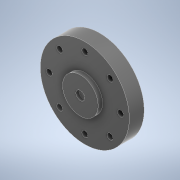
# Autodesk Inventor part: orczyk serwa okrągły 02-1
Saved by Autodesk Inventor 2021 (Build 250183000, 183)
## iProperties
Created: 2021-11-05
Part Number: orczyk serwa okrągły 02-1
Material: Generic
Document SubType Name: Modeling
Designer: Łukasz
Density: 1 g/cm^3
Appearance: Smooth - Black
Author: Łukasz
Autodesk Inventor part; units mm, degrees
ref_plane "YZ Plane" through (0, 0, 0) normal (1, 0, 0) x (0, 1, 0)
ref_plane "XZ Plane" through (0, 0, 0) normal (0, 1, 0) x (-1, 0, 0)
ref_plane "XY Plane" through (0, 0, 0) normal (0, 0, 1) x (1, 0, 0)
sketch "Sketch1" plane through (0, 0, 0) normal (0, 0, 1) x (1, 0, 0)
  circle A0 centre (0, 0) radius 15
  circle A1 centre (0, 12) radius 1
  circle A2 centre (-8.4853, 8.4853) radius 1
  circle A3 centre (-12, 0) radius 1
  circle A4 centre (-8.4853, -8.4853) radius 1
  circle A5 centre (0, -12) radius 1
  circle A6 centre (8.4853, -8.4853) radius 1
  circle A7 centre (12, 0) radius 1
  circle A8 centre (8.4853, 8.4853) radius 1
  circle A9 centre (0, 0) radius 1.5
  dimension "d0" = 30
  dimension "d1" = 2
  dimension "d4" = 360
  dimension "d6" = 12
  dimension "d9" = 3
  constraints: 10 centre point, 2 coincident, 17 other
  measures "d0" diameter of A0
  measures "d1" diameter of A1
  measures "d6" distance of point (0, 0) A1.centre
  measures "d9" diameter of A9
extrude "Extrusion1" add sketch "Sketch1" along normal blind 5
sketch "Sketch2" plane through (0, 0, 5) normal (0, 0, 1) x (1, 0, 0)
  point P0 (0, 0)
sketch "Sketch3" plane through (0, 0, 5) normal (0, 0, 1) x (1, 0, 0)
  circle A0 centre (0, 0) radius 6
  circle A1 centre (0, 0) radius 1.5 projected
  dimension "d10" = 12
  constraints: 1 centre point, 1 coincident
  measures "d10" diameter of A0
extrude "Extrusion2" add sketch "Sketch3" along normal blind 1.5
sketch "Sketch4" plane through (0, 0, 0) normal (0, 0, -1) x (-1, 0, 0)
  circle A0 centre (0, 0) radius 1.5 projected
  circle A1 centre (0, 0) radius 3.9
  dimension "d13" = 7.8
  constraints: 1 centre point, 1 coincident
  measures "d13" diameter of A1
extrude "Extrusion3" cut sketch "Sketch4" against normal blind 5.5
body "Solid1"
